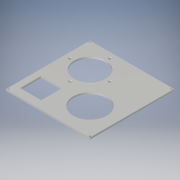
# Autodesk Inventor part: Housing_lid
Saved by Autodesk Inventor 2018 (Build 220112000, 112)
## iProperties
Created: 2021-04-22
Part Number: Housing_lid
Material: Aluminum 6061
Document SubType Name: Modeling
Designer: Ramana Bharathi
Mass: 301.79 g
Surface Area: 622.157 cm^2
Volume: 111.774 cm^3
Density: 2.7 g/cm^3
Appearance: Aluminum - Flat
Author: Ramana Bharathi
Autodesk Inventor part; units mm, degrees
ref_plane "YZ Plane" through (0, 0, 0) normal (1, 0, 0) x (0, 1, 0)
ref_plane "XZ Plane" through (0, 0, 0) normal (0, 1, 0) x (-1, 0, 0)
ref_plane "XY Plane" through (0, 0, 0) normal (0, 0, 1) x (1, 0, 0)
sketch "Sketch1" plane through (0, 0, 0) normal (0, 1, 0) x (-1, 0, 0)
  line L0 (0, 0) -> (200, 0)
  line L1 (200, 0) -> (200, -200)
  line L2 (200, -200) -> (0, -200)
  line L3 (0, -200) -> (0, 0)
  dimension "d0" = 200
  dimension "d1" = 200
  constraints: 8 end point, 2 parallel, 1 horizontal, 1 perpendicular
  measures "d0" distance of L1.end L2.end
  measures "d1" distance of L0.end L1.end
extrude "Extrusion1" add sketch "Sketch1" along normal blind 4
sketch "Sketch2" plane through (0, 4, 0) normal (0, 1, 0) x (1, 0, 0)
  circle A0 centre (-197, 197) radius 1.5
  line L0 (0, 200) -> (-200, 200)
  line L1 (-200, 200) -> (-200, 0)
  circle A1 centre (-197, 3) radius 1.5
  line L2 (-200, 0) -> (0, 0)
  circle A2 centre (-3, 197) radius 1.5
  line L3 (0, 0) -> (0, 200)
  circle A3 centre (-3, 3) radius 1.5
  dimension "d4" = 3
  dimension "d5" = 3
  dimension "d6" = 3
  dimension "d7" = 3
  dimension "d8" = 3
  dimension "d9" = 3
  dimension "d10" = 3
  dimension "d11" = 3
  dimension "d12" = 3
  dimension "d13" = 3
  dimension "d14" = 3
  dimension "d15" = 3
  constraints: 8 end point, 4 centre point
  measures "d4" diameter of A0
  measures "d5" distance from line of L0 A0.centre
  measures "d6" distance from line of L1 A0.centre
  measures "d7" diameter of A1
  measures "d8" distance from line of L1 A1.centre
  measures "d9" distance from line of L2 A1.centre
  measures "d10" diameter of A2
  measures "d11" distance from line of L0 A2.centre
  measures "d12" distance from line of L3 A2.centre
  measures "d13" diameter of A3
  measures "d14" distance from line of L3 A3.centre
  measures "d15" distance from line of L2 A3.centre
hole "Hole1" at (-197, 4, -197) at (-3, 4, -197) at (-197, 4, -3) at (-3, 4, -3) direction (0, -1, 0) diameter 3 end through all
sketch "Sketch3" plane through (0, 4, 0) normal (0, 1, 0) x (1, 0, 0)
  circle A0 centre (-65, 65) radius 40
  line L0 (0, 0) -> (0, 200) projected
  line L1 (-200, 0) -> (0, 0) projected
  circle A1 centre (-140, 140) radius 37.5
  line L2 (0, 200) -> (-200, 200) projected
  line L3 (-200, 200) -> (-200, 0) projected
  circle A2 centre (-140, 140) radius 55
  line L4 (-185, 78) -> (-135, 78)
  line L5 (-135, 78) -> (-135, 10)
  line L6 (-135, 10) -> (-185, 10)
  line L7 (-185, 10) -> (-185, 78)
  circle A3 centre (-65, 65) radius 50
  circle A4 centre (-65, 65) radius 60
  line L8 (-185, 19) -> (-135, 19)
  line L9 (-135, 19) -> (-135, 69)
  line L10 (-135, 69) -> (-185, 69)
  line L11 (-185, 69) -> (-185, 19)
  dimension "d23" = 80
  dimension "d24" = 65
  dimension "d25" = 65
  dimension "d26" = 75
  dimension "d29" = 140
  dimension "d30" = 140
  dimension "d31" = 110
  dimension "d32" = 50
  dimension "d33" = 68
  dimension "d34" = 10
  dimension "d59" = 100
  dimension "d60" = 120
  dimension "d61" = 135
  dimension "d62" = 50
  dimension "d63" = 50
  dimension "d64" = 9
  constraints: 16 end point, 5 centre point, 4 parallel, 3 coincident, 2 horizontal, 2 perpendicular, 1 point on line
  measures "d23" diameter of A0
  measures "d24" distance from line of L0 A0.centre
  measures "d25" distance from line of L1 A0.centre
  measures "d26" diameter of A1
  measures "d29" distance from line of L1 A1.centre
  measures "d30" distance from line of L0 A1.centre
  measures "d31" diameter of A2
  measures "d32" distance of L5.end L6.end
  measures "d33" distance of L4.end L5.end
  measures "d34" distance between parallel lines of L1 L6
  measures "d59" diameter of A3
  measures "d60" diameter of A4
  measures "d61" distance between parallel lines of L0 L5
  measures "d62" distance of L10.end L9.end
  measures "d63" distance of L9.end L8.end
  measures "d64" distance between parallel lines of L8 L6
extrude "Extrusion2" cut sketch "Sketch3" against normal through all contours A0 | A1 | L10 L5 L8 L7
sketch "Sketch4" plane through (0, 4, 0) normal (0, 1, 0) x (1, 0, 0)
  circle A0 centre (-140, 140) radius 37.5 projected
  circle A1 centre (-140, 140) radius 47.5
  circle A2 centre (-140, 187.5) radius 2
  circle A3 centre (-187.5, 140) radius 2
  circle A4 centre (-140, 92.5) radius 2
  circle A5 centre (-92.5, 140) radius 2
  point P0 (0, 0)
  dimension "d38" = 95
  dimension "d39" = 4
  dimension "d42" = 360
  constraints: 4 centre point, 1 coincident, 1 vertical alignment, 11 other
  measures "d39" diameter of A2
hole "Hole2" at (-187.5, 4, -140) at (-140, 4, -92.5) at (-140, 4, -187.5) at (-92.5, 4, -140) direction (0, -1, 0) diameter 4 end through all countersink diameter 8 countersink angle 90
thread "Thread1" size "M4x0.7" class "6H" standard "ANSI Metric M Profile" full length
thread "Thread2" size "M4x0.7" class "6H" standard "ANSI Metric M Profile" full length
thread "Thread3" size "M4x0.7" class "6H" standard "ANSI Metric M Profile" full length
thread "Thread4" size "M4x0.7" class "6H" standard "ANSI Metric M Profile" full length
thread "Thread5" size "M3x0.5" class "6H" standard "ANSI Metric M Profile" full length
thread "Thread6" size "M3x0.5" class "6H" standard "ANSI Metric M Profile" full length
thread "Thread7" size "M3x0.5" class "6H" standard "ANSI Metric M Profile" full length
thread "Thread8" size "M3x0.5" class "6H" standard "ANSI Metric M Profile" full length
fillet "Fillet1" radius 2 4 edges at (-185, 2, -69) (-185, 2, -19) (-135, 2, -69) (-135, 2, -19)
body "Solid1"
